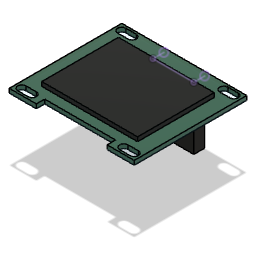
All together (Autodesk Fusion 360 archive; units mm, degrees)
design "oled"
description: IIC OLED 0.96" 4Pin SSD1306
part number: GME12864-11
Autodesk Fusion 360 part; units mm, degrees
sketch "Sketch1" plane through (0, 0, 0) normal (0, 1, 0) x (1, 0, 0)
  line L0 (0, 0) -> (30, 0)
  line L1 (30, 0) -> (30, -27)
  line L2 (30, -27) -> (0, -27)
  line L3 (0, -27) -> (0, 0)
  line L4 (6.5, -27) -> (6.5, -25)
  line L5 (6.5, -25) -> (23.5, -25)
  line L6 (23.5, -25) -> (23.5, -27)
  line L7 (15, -27) -> (15, -25) construction
  line L8 (3.5, -4.3) -> (26.5, -4.3)
  line L9 (26.5, -4.3) -> (26.5, -22.7)
  line L10 (26.5, -22.7) -> (3.5, -22.7)
  line L11 (3.5, -22.7) -> (3.5, -4.3)
  line L12 (1.5, -2.5) -> (4, -2.5)
  arc A0 (4, -2.5) -> (4, -0.5) centre (4, -1.5) ccw
  line L13 (4, -0.5) -> (1.5, -0.5)
  arc A1 (1.5, -0.5) -> (1.5, -2.5) centre (1.5, -1.5) ccw
  line L14 (1.5, -1.5) -> (4, -1.5) construction
  line L15 (15, 0) -> (15, -25) construction
  line L16 (0, -13.5) -> (30, -13.5) construction
  arc A2 (26, -0.5) -> (26, -2.5) centre (26, -1.5) ccw
  line L17 (26, -0.5) -> (28.5, -0.5)
  arc A3 (28.5, -2.5) -> (28.5, -0.5) centre (28.5, -1.5) ccw
  line L18 (28.5, -2.5) -> (26, -2.5)
  line L19 (26, -26.5) -> (28.5, -26.5)
  arc A4 (28.5, -26.5) -> (28.5, -24.5) centre (28.5, -25.5) ccw
  line L20 (28.5, -24.5) -> (26, -24.5)
  arc A5 (26, -24.5) -> (26, -26.5) centre (26, -25.5) ccw
  line L21 (4, -26.5) -> (1.5, -26.5)
  arc A6 (4, -26.5) -> (4, -24.5) centre (4, -25.5) ccw
  arc A7 (1.5, -24.5) -> (1.5, -26.5) centre (1.5, -25.5) ccw
  line L22 (1.5, -24.5) -> (4, -24.5)
  dimension "d1" = 30
  dimension "d2" = 27
  dimension "d3" = 6.5
  dimension "d4" = 2
  dimension "d5" = 3.5
  dimension "d6" = 3.5
  dimension "d7" = 4.3
  dimension "d8" = 4.3
  dimension "d22" = 1.5
  dimension "d23" = 1.5
  dimension "d24" = 1
  dimension "d25" = 2.5
  constraint horizontal L0
  constraint vertical L1
  constraint horizontal L2
  constraint vertical L3
  constraint coincident L0.start L3.end
  constraint coincident L2 L4.start
  constraint perpendicular L2 L4
  constraint perpendicular L4 L5
  constraint coincident L2 L6.end
  constraint perpendicular L2 L6
  constraint midpoint L2 L7.start
  constraint midpoint L5 L7.end
  constraint perpendicular L2 L7
  constraint horizontal L8
  constraint vertical L9
  constraint horizontal L10
  constraint vertical L11
  constraint tangent L12 A0
  constraint tangent A0 L13
  constraint parallel L12 L13
  constraint tangent L13 A1
  constraint tangent L12 A1
  constraint horizontal L14
  constraint midpoint L0 L15.start
  constraint midpoint L3 L16.start
  constraint midpoint L1 L16.end
  constraint symmetric L12.start L15 A3.start
  constraint symmetric L12.end L15 A2.end
  constraint symmetric A0.end L15 A2.start
  constraint symmetric L13.end L15 L17.end
  constraint symmetric A0 L15 A2
  constraint symmetric A1 L15 A3
  constraint symmetric L12.start L16 A7.start
  constraint symmetric L12.end L16 A6.end
  constraint symmetric A0.end L16 L21.start
  constraint symmetric L13.end L16 L21.end
  constraint symmetric A0 L16 A6
  constraint symmetric A1 L16 A7
  constraint symmetric L16 A2.end L20.end
  constraint symmetric L16 A2.start L19.start
  constraint symmetric L16 A2 A5
  constraint symmetric L16 L17.end L19.end
  constraint symmetric L16 A3.start A4.end
  constraint symmetric L16 A3 A4
  measures "d1" distance of L0.start L0.end
  measures "d2" distance of L0.start L2.end
  measures "d3" distance of L1 L6
  measures "d4" distance of L2 L5
  measures "d5" distance of L1 L9
  measures "d6" distance of L3 L11
  measures "d7" distance of L0 L8
  measures "d8" distance of L2 L10
  measures "d22" distance of L3 A1.centre
  measures "d23" distance of L0 A1.centre
  measures "d24" radius of A1
  measures "d25" distance of A1.centre A0.centre
extrude "Extrude1" add sketch "Sketch1" along normal blind 1 contours L8 L9 L10 L11 makes body 1
extrude "Extrude2" add sketch "Sketch1" against normal blind 1 separate body contours L0 L1 L2 L3 L4 L5 L6 | L8 L9 L10 L11 makes body 2
sketch "Sketch2" plane through (0, -1, 0) normal (0, -1, 0) x (1, 0, 0)
  line L0 (6.5, 25) -> (6.5, 27)
  line L1 (6.5, 27) -> (0, 27)
  line L2 (0, 27) -> (0, 0)
  line L3 (0, 0) -> (30, 0)
  line L4 (30, 0) -> (30, 27)
  line L5 (30, 27) -> (23.5, 27)
  line L6 (23.5, 27) -> (23.5, 25)
  line L7 (23.5, 25) -> (6.5, 25)
  line L8 (10.1, 2.6) -> (19.9, 2.6)
  line L9 (19.9, 2.6) -> (19.9, 0)
  line L10 (10.1, 0) -> (10.1, 2.6)
  line L11 (15, 0) -> (15, 2.6) construction
  arc A0 (26, 2.5) -> (26, 0.5) centre (26, 1.5) ccw
  line L12 (26, 2.5) -> (28.5, 2.5)
  arc A1 (28.5, 0.5) -> (28.5, 2.5) centre (28.5, 1.5) ccw
  line L13 (28.5, 0.5) -> (26, 0.5)
  arc A2 (26, 26.5) -> (26, 24.5) centre (26, 25.5) ccw
  line L14 (26, 26.5) -> (28.5, 26.5)
  arc A3 (28.5, 24.5) -> (28.5, 26.5) centre (28.5, 25.5) ccw
  line L15 (28.5, 24.5) -> (26, 24.5)
  arc A4 (4, 24.5) -> (4, 26.5) centre (4, 25.5) ccw
  line L16 (4, 24.5) -> (1.5, 24.5)
  arc A5 (1.5, 26.5) -> (1.5, 24.5) centre (1.5, 25.5) ccw
  line L17 (1.5, 26.5) -> (4, 26.5)
  arc A6 (1.5, 2.5) -> (1.5, 0.5) centre (1.5, 1.5) ccw
  line L18 (1.5, 2.5) -> (4, 2.5)
  arc A7 (4, 0.5) -> (4, 2.5) centre (4, 1.5) ccw
  line L19 (4, 0.5) -> (1.5, 0.5)
  dimension "d13" = 9.8
  dimension "d14" = 2.6
  constraint horizontal L8
  constraint vertical L9
  constraint vertical L10
  constraint midpoint L3 L11.start
  constraint perpendicular L3 L11
  constraint coincident L3 L9.end
  constraint coincident L3 L10.start
  constraint midpoint L8 L11.end
  measures "d13" distance of L8.start L8.end
  measures "d14" distance of L8.start L10.start
extrude "Extrude3" add sketch "Sketch2" along normal blind 15 separate body contours L3 L8 L9 L10 makes body 3
sketch "Minimal Projection" plane through (0, -1, 0) normal (0, -1, 0) x (1, 0, 0)
  arc A0 (26, 2.5) -> (26, 0.5) centre (26, 1.5) ccw
  line L0 (26, 2.5) -> (28.5, 2.5)
  arc A1 (28.5, 0.5) -> (28.5, 2.5) centre (28.5, 1.5) ccw
  line L1 (28.5, 0.5) -> (26, 0.5)
  arc A2 (26, 26.5) -> (26, 24.5) centre (26, 25.5) ccw
  line L2 (26, 26.5) -> (28.5, 26.5)
  arc A3 (28.5, 24.5) -> (28.5, 26.5) centre (28.5, 25.5) ccw
  line L3 (28.5, 24.5) -> (26, 24.5)
  arc A4 (4, 24.5) -> (4, 26.5) centre (4, 25.5) ccw
  line L4 (4, 24.5) -> (1.5, 24.5)
  arc A5 (1.5, 26.5) -> (1.5, 24.5) centre (1.5, 25.5) ccw
  line L5 (1.5, 26.5) -> (4, 26.5)
  arc A6 (1.5, 2.5) -> (1.5, 0.5) centre (1.5, 1.5) ccw
  line L6 (1.5, 2.5) -> (4, 2.5)
  arc A7 (4, 0.5) -> (4, 2.5) centre (4, 1.5) ccw
  line L7 (4, 0.5) -> (1.5, 0.5)
  line L8 (6.5, 25) -> (6.5, 27)
  line L9 (6.5, 27) -> (0, 27)
  line L10 (0, 27) -> (0, 0)
  line L11 (0, 0) -> (30, 0)
  line L12 (30, 0) -> (30, 27)
  line L13 (30, 27) -> (23.5, 27)
  line L14 (23.5, 27) -> (23.5, 25)
  line L15 (23.5, 25) -> (6.5, 25)
  line L16 (19.9, 0) -> (19.9, 2.6)
  line L17 (19.9, 2.6) -> (10.1, 2.6)
  line L18 (10.1, 2.6) -> (10.1, 0)

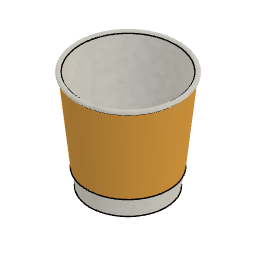
design "Cup"
Autodesk Fusion 360 part; units mm, degrees
sketch "Sketch3" plane through (0, 0, 0) normal (0, 1, 0) x (1, 0, 0)
  line L0 (0, 0) -> (22.3917, 0)
  line L1 (29, -54.5) -> (22.5, 5.5)
  line L2 (0, 5.5) -> (0, -54.5)
  line L3 (21.7959, 5.5) -> (28.2959, -54.5)
  line L4 (28.2959, -54.5) -> (29, -54.5)
  line L5 (21.7959, 5.5) -> (22.5, 5.5)
  line L6 (0, -0.7) -> (22.4676, -0.7)
  circle A0 centre (29.4178, -53.25) radius 1.25
  line L7 (29, -54.5) -> (29.4178, -54.5)
  line L8 (29.4333, -52.0001) -> (24.3174, -4.7764)
  line L9 (24.3174, -4.7764) -> (23.6214, -4.8518)
  arc A1 (22.5338, 5.1877) -> (21.8379, 5.1123) centre (22.1859, 5.15) ccw
  dimension "d4" = 60
  dimension "d5" = 58
  dimension "d6" = 45
  dimension "d7" = 5.5
  dimension "d9" = 0.7
  dimension "d10" = 0.7
  dimension "d11" = 2.5
  dimension "d12" = 47.5
  dimension "d13" = 0.7
  constraint coincident L0.start origin
  constraint horizontal L0
  constraint perpendicular L0 L2
  constraint coincident L0.start L2
  constraint horizontal L1.end L2.start
  constraint horizontal L1.start L2.end
  constraint horizontal L5
  constraint horizontal L4
  constraint coincident L0.end L3
  constraint parallel L1 L3
  constraint coincident L2 L6.start
  constraint coincident L3 L6.end
  constraint perpendicular L2 L6
  constraint tangent L3 A0
  constraint tangent L4 A0
  constraint coincident A0 L7.end
  constraint tangent A0 L7
  constraint coincident A0 L8.start
  constraint parallel L1 L8
  constraint coincident L1 L9.end
  constraint perpendicular L1 L9
  constraint coincident L3 A1.end
  constraint coincident L1 A1.start
  constraint tangent L1 A1
  constraint tangent L3 A1
  constraint tangent L5 A1
  measures "d4" distance of L2.start L2.end
  measures "d7" distance of L0 L5
  measures "d9" distance of L1 L3
  measures "d10" distance of L0 L6
  measures "d11" diameter of A0
  measures "d12" distance of L8.start L8.end
  measures "d13" distance of L8.end L9.end
revolve "Revolve1" add sketch "Sketch3" angle 360 about axis through (0, 0, -5.5) along (0, 0, 1) contours L0 L2 L3 L6 | L1 L3 A0 A1 | L1 A0 | L1 A0 makes body 1
revolve "Revolve2" add sketch "Sketch3" angle 360 about axis through (0, 0, -5.5) along (0, 0, 1) separate body contours L1 A0 L8 L9 makes body 2
equation "d10 = d9"

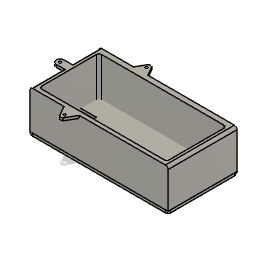
design "Sensor Housing"
Autodesk Fusion 360 part; units mm, degrees
sketch "Outside box sketch" plane through (0, 0, 0) normal (0, 0, 1) x (1, 0, 0)
  line L0 (1, 0) -> (52, 0)
  line L1 (53, 1) -> (53, 14.9)
  line L2 (52, 15.9) -> (1, 15.9)
  line L3 (0, 14.9) -> (0, 1)
  arc A0 (1, 15.9) -> (0, 14.9) centre (1, 14.9) ccw
  arc A1 (0, 1) -> (1, 0) centre (1, 1) ccw
  arc A2 (53, 14.9) -> (52, 15.9) centre (52, 14.9) ccw
  arc A3 (52, 0) -> (53, 1) centre (52, 1) ccw
  point P0 (53, 0)
  point P1 (0, 15.9)
  dimension "d1" = 53
  dimension "d2" = 15.9
  dimension "d13" = 1
  dimension "d14" = 1
  dimension "d15" = 1
  dimension "d16" = 1
  constraint horizontal L0
  constraint vertical L1
  constraint horizontal L2
  constraint vertical L3
  constraint coincident P1 L2
  constraint coincident P1 L3
  constraint tangent L2 A0
  constraint tangent L3 A0
  constraint coincident origin L0
  constraint coincident origin L3
  constraint tangent L0 A1
  constraint tangent L3 A1
  constraint tangent L2 A2
  constraint tangent L1 A2
  constraint coincident P0 L0
  constraint coincident P0 L1
  constraint tangent L0 A3
  constraint tangent L1 A3
  measures "d1" distance of origin P0
  measures "d2" distance of origin P1
  measures "d13" radius of A0
  measures "d14" radius of A1
  measures "d15" radius of A2
  measures "d16" radius of A3
extrude "Extrude1" add sketch "Outside box sketch" along normal blind 26.5 makes body 1
sketch "Hole sketch" plane through (0, 0, 0) normal (0, 1, 0) x (1, 0, 0)
  line L0 (3, -2) -> (50, -2)
  line L1 (51, -3) -> (51, -24)
  line L2 (50, -25) -> (3, -25)
  line L3 (2, -24) -> (2, -3)
  arc A0 (3, -2) -> (2, -3) centre (3, -3) ccw
  arc A1 (51, -3) -> (50, -2) centre (50, -3) ccw
  arc A2 (50, -25) -> (51, -24) centre (50, -24) ccw
  arc A3 (2, -24) -> (3, -25) centre (3, -24) ccw
  dimension "d17" = 1
  constraint horizontal L0
  constraint vertical L1
  constraint horizontal L2
  constraint vertical L3
  constraint tangent L0 A0
  constraint tangent L3 A0
  constraint tangent L0 A1
  constraint tangent L1 A1
  constraint equal A0 A1
  constraint tangent L1 A2
  constraint tangent L2 A2
  constraint equal A0 A2
  constraint tangent L2 A3
  constraint tangent L3 A3
  constraint equal A0 A3
  measures "d17" radius of A0
extrude "Extrude2" cut sketch "Hole sketch" along normal blind 25 bodies 1
sketch "Base sketch" plane through (0, 0, 0) normal (0, 1, 0) x (1, 0, 0)
  line L0 (1, 0) -> (52, 0)
  line L1 (53, -1) -> (53, -25.5)
  line L2 (52, -26.5) -> (1, -26.5)
  arc A0 (1, 0) -> (0, -1) centre (1, -1) ccw
  arc A1 (53, -1) -> (52, 0) centre (52, -1) ccw
  arc A2 (52, -26.5) -> (53, -25.5) centre (52, -25.5) ccw
  arc A3 (0, -25.5) -> (1, -26.5) centre (1, -25.5) ccw
  line L3 (0, -1) -> (0, -25.5)
  line L4 (1, -9) -> (8, -9)
  line L5 (8, -9) -> (8, -18)
  line L6 (8, -18) -> (1, -18)
  line L7 (1, -18) -> (1, -9)
  line L8 (1, -9) -> (8, -9)
  line L9 (1, -9) -> (8, -9)
  line L10 (8, -9) -> (8, -18)
  line L11 (45, -9) -> (45, -18)
  line L12 (52, -9) -> (45, -9)
  line L13 (52, -18) -> (52, -9)
  line L14 (45, -18) -> (52, -18)
  point P0 (53, 0)
  point P1 (0, -26.5)
  constraint horizontal L0
  constraint vertical L1
  constraint horizontal L2
  constraint coincident origin L0
  constraint tangent L0 A0
  constraint coincident P0 L0
  constraint coincident P0 L1
  constraint tangent L0 A1
  constraint tangent L1 A1
  constraint tangent L1 A2
  constraint tangent L2 A2
  constraint equal A1 A2
  constraint coincident P1 L2
  constraint tangent L2 A3
  constraint equal A1 A3
  constraint vertical L3
  constraint horizontal L4
  constraint vertical L5
  constraint horizontal L6
  constraint vertical L7
  constraint horizontal L8
  constraint horizontal L9
  constraint vertical L10
extrude "Extrude3" add sketch "Base sketch" along normal blind 1 separate body contours L0 L1 L2 A0 A1 A2 A3 L3 | L4 L5 L6 L7 L8 L9 L10 | L11 L12 L13 L14 makes body 2
extrude "Extrude4" cut sketch "Base sketch" along normal blind 26 contours L0 L1 L2 A0 A1 A2 A3 L3 | L4 L5 L6 L7 L8 L9 L10 | L11 L12 L13 L14 bodies 2
extrude "Extrude5" add sketch "Base sketch" along normal blind 1 bodies 2
sketch "Front hole sketch" plane through (0, 0, 0) normal (0, 1, 0) x (1, 0, 0)
  line L0 (-2.4094, -14) -> (0, -14)
  line L1 (0, -14) -> (0, -11)
  line L2 (0, -11) -> (-2.4095, -11)
  arc A0 (-2.4095, -11) -> (-2.4094, -14) centre (-2.4095, -12.5) ccw
  circle A1 centre (-2.4095, -12.5) radius 0.5
  dimension "d24" = 1
  constraint horizontal L0
  constraint vertical L1
  constraint horizontal L2
  constraint concentric A0 A1
  measures "d24" diameter of A1
extrude "Extrude6" add sketch "Front hole sketch" along normal blind 13.9 separate body makes body 3
extrude "Extrude7" cut 1 faces at (-0.6365, 0, 12.5) along direction (0, 1, 0) blind 12.9 on bodies 3 bodies 3
sketch "Side holes sketch" plane through (0, 0, 0) normal (0, 1, 0) x (1, 0, 0)
  line L0 (13.1017, 0.0509) -> (19, 0.0509) construction
  line L1 (13.1017, 0.0509) -> (18.8983, 0.0509)
  line L2 (13.1017, -26.6022) -> (18.8983, -26.6022)
  line L3 (13.1017, -26.6022) -> (15.3819, -30.5516)
  line L4 (16, -31.6222) -> (16.1017, -31.7984)
  line L5 (18.8983, -26.6022) -> (16.6709, -30.4601)
  line L6 (16, -31.6222) -> (15.8983, -31.7984)
  arc A0 (15.3819, -30.5516) -> (16.6709, -30.4601) centre (15.9305, -29.1556) ccw
  circle A1 centre (15.9305, -29.1556) radius 0.5
  line L7 (18.7811, -0.0196) -> (16.6709, 3.6353)
  line L8 (13.2189, -0.0196) -> (15.3819, 3.7269)
  line L9 (13.2189, -0.0196) -> (18.7811, -0.0196)
  arc A2 (16.6709, 3.6353) -> (15.3819, 3.7269) centre (15.9305, 2.3308) ccw
  circle A3 centre (15.9305, 2.3308) radius 0.5
  point P0 (15.9305, 2.3308)
  dimension "d32" = 1
  dimension "d33" = 1
  constraint horizontal L0
  constraint coincident L4.start L5
  constraint collinear L3 L4
  constraint collinear L5 L6
  constraint concentric A0 A1
  constraint concentric A2 A3
  measures "d32" diameter of A1
  measures "d33" diameter of A3
extrude "Extrude8" add sketch "Side holes sketch" along normal blind 13.9 separate body contours L1 L7 L8 A2 | L2 L3 L5 A0 makes body 4 at (15.0865, 4.6333, -0.0509) makes body 5 at (15.0339, 4.6333, 26.6022)
extrude "Extrude9" cut 2 faces at (15.9893, 0, 27.2871) (15.9893, 0, -0.6446) along direction (0, 1, 0) blind 12.9 on bodies 4 5 bodies 4 5
extrude "Extrude10" add 2 faces at (15.9893, 13.9, 27.2871) (15.9893, 13.9, -0.6446) along direction (0, 1, 0) blind 2 on bodies 4 5 bodies 5 4
extrude "Extrude11" cut 2 faces at (15.9893, 12.9, 27.2871) (15.9893, 12.9, -0.6446) along direction (0, 1, 0) blind 2 on bodies 4 5 bodies 4 5
extrude "Extrude12" add 1 faces at (-0.6365, 13.9, 12.5) along direction (0, 1, 0) blind 2 on bodies 3 bodies 1 2 3
extrude "Extrude13" cut 1 faces at (-0.6365, 12.9, 12.5) along direction (0, 1, 0) blind 2 on bodies 1 bodies 1
extrude "Extrude14" add 1 faces at (0, 15.2333, 13) along direction (1, 0, 0) blind 1 on bodies 1 bodies 1
extrude "Extrude15" add 1 faces at (15.0865, 15.2333, -0.0509) along direction (0, 0, 1) blind 2 on bodies 4 bodies 1 4
extrude "Extrude16" add 1 faces at (15.0339, 15.2333, 26.6022) along direction (0, 0, -1) blind 1.6 on bodies 5 bodies 1 5
named bodies: "Outside box", "Base", "Front hole", "Side hole 1", "Side hole 2"

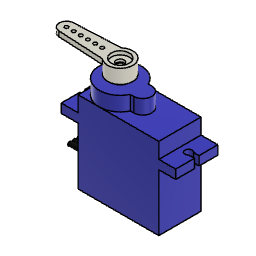
design "SG90 Micro Servo"
Autodesk Fusion 360 part; units mm, degrees
sketch "Sketch2" plane through (0, 0, 0) normal (0, 1, 0) x (1, 0, 0)
  line L0 (0, 0) -> (22.5, 0)
  line L1 (22.5, 0) -> (22.5, -22.75)
  line L2 (22.5, -22.75) -> (0, -22.75)
  line L3 (0, -22.75) -> (0, 0)
  line L4 (-4.7, -15.9) -> (-4.7, -18.4)
  line L5 (27.2, -18.4) -> (27.2, -15.9)
  line L6 (-4.7, -18.4) -> (0, -18.4)
  line L7 (22.5, -18.4) -> (27.2, -18.4)
  line L8 (27.2, -15.9) -> (22.5, -15.9)
  line L9 (0, -15.9) -> (-4.7, -15.9)
  dimension "d3" = 22.5
  dimension "d4" = 22.75
  dimension "d6" = 4.35
  dimension "d7" = 2.5
  dimension "d8" = 4.7
  dimension "d9" = 4.7
  constraint horizontal L0
  constraint vertical L1
  constraint horizontal L2
  constraint vertical L3
  constraint coincident L0.start L3.end
  constraint horizontal L8
  constraint vertical L4
  constraint horizontal L6
  constraint vertical L5
  constraint coincident L3 L6.end
  constraint coincident L1 L7.start
  constraint collinear L6 L7
  constraint coincident L1 L8.end
  constraint coincident L3 L9.start
  constraint collinear L8 L9
  measures "d3" distance of L0.start L0.end
  measures "d4" distance of L0.start L2.end
  measures "d6" distance of L2 L6
  measures "d7" distance of L5.end L5.start
  measures "d8" distance of L1 L5
  measures "d9" distance of L3 L4
extrude "Extrude2" add sketch "Sketch2" along normal blind 11.75 makes body 1
sketch "Sketch3" plane through (0, 0, 22.75) normal (0, 0, 1) x (-1, 0, 0)
  line L0 (0, 0) -> (-22.5, 0)
  line L1 (-22.5, 0) -> (-22.5, -11.75)
  line L2 (-22.5, -11.75) -> (0, -11.75)
  line L3 (0, -11.75) -> (0, 0)
  circle A0 centre (-5.875, -5.875) radius 5.875
  line L4 (-5.875, -5.875) -> (-12.175, -5.875) construction
  line L5 (-11.1915, -8.375) -> (-12.175, -8.375)
  line L6 (-11.1915, -3.375) -> (-12.175, -3.375)
  arc A1 (-12.175, -3.375) -> (-12.175, -8.375) centre (-12.175, -5.875) ccw
  dimension "d13" = 6.3
  dimension "d14" = 2.5
  constraint tangent L0 A0
  constraint tangent L2 A0
  constraint tangent L3 A0
  constraint coincident A0.centre L4.start
  constraint coincident L4.end A1.centre
  constraint horizontal L4
  constraint coincident A0 L5.start
  constraint tangent L5 A1
  constraint coincident A0 L6.start
  constraint tangent L6 A1
  constraint horizontal L5
  constraint horizontal L6
  measures "d13" distance of A0.centre L4.end
  measures "d14" radius of A1
extrude "Extrude3" add sketch "Sketch3" along normal blind 4 contours A0 | A0 L5 L6 A1 bodies 1
sketch "Sketch4" plane through (0, 0, 26.75) normal (0, 0, 1) x (-1, 0, 0)
  arc A0 (-11.1915, -8.375) -> (-11.1915, -3.375) centre (-5.875, -5.875) ccw
  line L0 (-11.1915, -3.375) -> (-12.175, -3.375)
  arc A1 (-12.175, -3.375) -> (-12.175, -8.375) centre (-12.175, -5.875) ccw
  line L1 (-12.175, -8.375) -> (-11.1915, -8.375)
  circle A2 centre (-5.875, -5.875) radius 2.3
  circle A3 centre (-5.875, -5.875) radius 0.75
  dimension "d17" = 4.6
  dimension "d28" = 1.5
  constraint concentric A0 A2
  constraint concentric A2 A3
  measures "d17" diameter of A2
  measures "d28" diameter of A3
extrude "Extrude4" add sketch "Sketch4" along normal blind 3.15 separate body contours A2 makes body 2
sketch "Sketch5" plane through (0, 0, 18.4) normal (0, 0, 1) x (-1, 0, 0)
  line L0 (4.7, 0) -> (0, 0)
  line L1 (0, 0) -> (0, -11.75)
  line L2 (0, -11.75) -> (4.7, -11.75)
  line L3 (4.7, -11.75) -> (4.7, 0)
  line L4 (-22.5, 0) -> (-27.2, 0)
  line L5 (-27.2, 0) -> (-27.2, -11.75)
  line L6 (-27.2, -11.75) -> (-22.5, -11.75)
  line L7 (-22.5, -11.75) -> (-22.5, 0)
  line L8 (-27.2, -5.875) -> (4.7, -5.875) construction
  line L9 (-11.25, -5.875) -> (-11.25, -0.3179)
  line L10 (4.7, -6.525) -> (3.1599, -6.525)
  line L11 (4.7, -5.225) -> (3.1599, -5.225)
  arc A0 (3.1599, -5.225) -> (3.1599, -6.525) centre (2.4, -5.875) ccw
  arc A1 (-25.6599, -6.525) -> (-25.6599, -5.225) centre (-24.9, -5.875) ccw
  line L12 (-27.2, -5.225) -> (-25.6599, -5.225)
  line L13 (-27.2, -6.525) -> (-25.6599, -6.525)
  dimension "d20" = 2
  dimension "d21" = 1.3
  dimension "d22" = 2.3
  constraint midpoint L5 L8.start
  constraint midpoint L3 L8.end
  constraint midpoint L8 L9.start
  constraint perpendicular L8 L9
  constraint coincident L8 A0.centre
  constraint coincident L3 L10.start
  constraint perpendicular L3 L10
  constraint coincident L3 L11.start
  constraint perpendicular L3 L11
  constraint symmetric L8 L10 L11
  constraint symmetric L9 L10.start L13.start
  constraint symmetric L9 L10.end A1.start
  constraint symmetric L9 L11.start L12.start
  constraint symmetric L9 L11.end A1.end
  constraint symmetric L9 A0 A1
  measures "d20" diameter of A0
  measures "d21" distance of L10 L11
  measures "d22" distance of L3 A0.centre
extrude "Extrude5" cut sketch "Sketch5" against normal through all contours L3 L10 L11 A0 | L5 A1 L12 L13 bodies 1
sketch "Sketch6" plane through (0, 0, 0) normal (-1, 0, 0) x (0, -1, 0)
  line L0 (0, 0) -> (0, 15.9)
  line L1 (0, 15.9) -> (-11.75, 15.9)
  line L2 (-11.75, 15.9) -> (-11.75, 0)
  line L3 (-11.75, 0) -> (0, 0)
  line L4 (-4.075, 5.7) -> (-7.675, 5.7) construction
  line L5 (-7.675, 5.7) -> (-7.675, 4.5) construction
  line L6 (-7.675, 4.5) -> (-4.075, 4.5) construction
  line L7 (-4.075, 4.5) -> (-4.075, 5.7) construction
  line L8 (-5.875, 4.5) -> (-5.875, 0) construction
  circle A0 centre (-5.875, 5.1) radius 0.6
  circle A1 centre (-4.675, 5.1) radius 0.6
  circle A2 centre (-7.075, 5.1) radius 0.6
  dimension "d24" = 1.2
  dimension "d25" = 4.5
  constraint horizontal L4
  constraint vertical L5
  constraint horizontal L6
  constraint vertical L7
  constraint midpoint L6 L8.start
  constraint coincident L3 L8.end
  constraint perpendicular L3 L8
  constraint midpoint L3 L8.end
  constraint tangent L4 A0
  constraint coincident L8.start A0
  constraint tangent L4 A1
  constraint tangent L7 A1
  constraint tangent L6 A1
  constraint tangent L4 A2
  constraint tangent L5 A2
  constraint tangent L6 A2
  constraint tangent A0 A1
  constraint tangent A0 A2
  measures "d24" distance of L4.start L6.end
  measures "d25" distance of L8.start L8.end
extrude "Extrude6" add sketch "Sketch6" along normal blind 7 separate body contours A0 | A2 | A1 makes body 3
sketch "Sketch1" plane through (0, 0, 29.9) normal (0, 0, 1) x (-1, 0, 0) in component "Horn"
  circle A0 centre (-5.875, -5.875) radius 0.75
  circle A1 centre (-5.875, -5.875) radius 2.3
  circle A2 centre (-5.875, -5.875) radius 3.5
  circle A3 centre (-5.875, -5.875) radius 2.5
  line L0 (-3.5886, -8.525) -> (9.2267, -7.8724)
  line L1 (-3.5886, -3.225) -> (9.2267, -3.8776)
  arc A4 (9.2267, -7.8724) -> (9.2267, -3.8776) centre (9.125, -5.875) ccw
  line L2 (-5.875, -5.875) -> (9.125, -5.875) construction
  circle A5 centre (9.125, -5.875) radius 0.5
  circle A6 centre (7.125, -5.875) radius 0.5
  circle A7 centre (5.125, -5.875) radius 0.5
  circle A8 centre (3.125, -5.875) radius 0.5
  circle A9 centre (1.125, -5.875) radius 0.5
  circle A10 centre (-0.875, -5.875) radius 0.5
  circle A11 centre (-5.875, -5.875) radius 1.1
  dimension "d29" = 7
  dimension "d30" = -1
  dimension "d32" = 2
  dimension "d33" = 5.3
  dimension "d34" = 1
  dimension "d37" = -10
  dimension "d38" = 0
  dimension "d39" = 15
  dimension "d42" = 2.2
  constraint concentric A0 A2
  constraint coincident A2 L0.start
  constraint coincident A2 L1.start
  constraint tangent L0 A4
  constraint tangent L1 A4
  constraint coincident A0.centre A1.centre
  constraint coincident A4.centre L2.end
  constraint horizontal L2
  constraint symmetric L0.start L1.start L2
  constraint concentric A4 A5
  constraint concentric A2 A11
  measures "d29" diameter of A2
  measures "d32" radius of A4
  measures "d33" vertical distance of L0.start L1.start
  measures "d34" diameter of A5
  measures "d39" distance of A0.centre A4.centre
  measures "d42" diameter of A11
extrude "Extrude1" add sketch "Sketch1" against normal blind 2.2 separate body contours A2 | A3 makes body 4 in component "Horn"
extrude "Extrude2'" add sketch "Sketch1" along normal blind 1.7 contours A2 bodies 4 in component "Horn"
extrude "Extrude3'" add sketch "Sketch1" against normal blind 1.4 from surface at 1.7 contours A2 L0 L1 A4 bodies 4 in component "Horn"
extrude "Extrude4'" add sketch "Sketch1" along normal up to surface (0.7 mm away) contours A1 | A3 bodies 4 in component "Horn"
component "Horn" placed x (1, 0, 0) y (0, 1, 0) z (0, 0, 1) at (0, 0, 0)
equation "d43 = 3.9 mm - 2.2 mm"
named bodies: "Body", "Wires", "Mount"

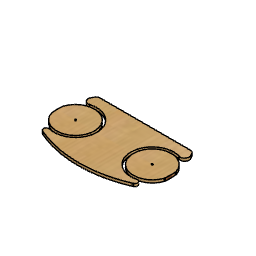
design "Cup Holder"
Autodesk Fusion 360 part; units mm, degrees
sketch "Sketch1" plane through (0, 0, 3) normal (0, 0, 1) x (-1, 0, 0)
  line L0 (27.1642, 47.5117) -> (28.8849, 49.9691)
  line L1 (28.8849, 49.9691) -> (37.0764, 44.2334)
  line L2 (37.0764, 44.2334) -> (35.3557, 41.7759)
  line L3 (35.3557, 41.7759) -> (27.1642, 47.5117)
  line L4 (-28.8849, 49.9691) -> (-27.1642, 47.5117)
  line L5 (-27.1642, 47.5117) -> (-35.3557, 41.7759)
  line L6 (-35.3557, 41.7759) -> (-37.0764, 44.2334)
  line L7 (-37.0764, 44.2334) -> (-28.8849, 49.9691)
  circle A0 centre (0, 0) radius 62.5
  line L8 (-45, -37.5) -> (-45, -34.5)
  line L9 (-45, -34.5) -> (-27, -34.5)
  line L10 (-27, -34.5) -> (-27, -37.5)
  line L11 (-27, -37.5) -> (-45, -37.5)
  line L12 (-9, -37.5) -> (-9, -34.5)
  line L13 (-9, -34.5) -> (9, -34.5)
  line L14 (9, -34.5) -> (9, -37.5)
  line L15 (9, -37.5) -> (-9, -37.5)
  line L16 (27, -37.5) -> (27, -34.5)
  line L17 (27, -34.5) -> (45, -34.5)
  line L18 (45, -34.5) -> (45, -37.5)
  line L19 (45, -37.5) -> (27, -37.5)
  circle A1 centre (-42.2822, 0) radius 21.8379 construction
  circle A2 centre (-42.2822, 0) radius 22.5338 construction
  circle A3 centre (-42.2822, 0) radius 20.8379
  circle A4 centre (-42.2822, 0) radius 23.5338
  line L20 (-45, -34.5) -> (-50, -34.5)
  line L21 (-50, -34.5) -> (-45, -34.5)
  line L22 (-45, -34.5) -> (-27, -34.5)
  line L23 (-27, -34.5) -> (-9, -34.5)
  line L24 (-9, -34.5) -> (9, -34.5)
  line L25 (9, -34.5) -> (27, -34.5)
  line L26 (27, -34.5) -> (45, -34.5)
  line L27 (45, -34.5) -> (50, -34.5)
  line L28 (50, -34.5) -> (45, -34.5)
  line L29 (45, -34.5) -> (27, -34.5)
  line L30 (27, -34.5) -> (9, -34.5)
  line L31 (9, -34.5) -> (-9, -34.5)
  line L32 (-9, -34.5) -> (-27, -34.5)
  line L33 (-27, -34.5) -> (-45, -34.5)
  arc A5 (-53.2887, -32.6583) -> (-50, -34.5) centre (-50, -30.6429) ccw
  arc A6 (50, -34.5) -> (53.2887, -32.6583) centre (50, -30.6429) ccw
  arc A7 (49.0193, 28.9228) -> (-49.0193, 28.9228) centre (0, -86.0646) ccw
  arc A8 (-49.0193, 28.9228) -> (-60.5532, 15.4777) centre (-41.1762, 10.5248) ccw
  arc A9 (60.5532, 15.4777) -> (49.0193, 28.9228) centre (41.1762, 10.5248) ccw
  line L34 (0, 0) -> (0, -86.0646) construction
  line L35 (-43.5472, 36.0401) -> (-35.3557, 41.7759) construction
  circle A10 centre (42.2822, 0) radius 23.5338
  circle A11 centre (42.2822, 0) radius 20.8379
  circle A12 centre (-42.2822, 0) radius 1
  circle A13 centre (42.2822, 0) radius 1
  line L36 (-39.2873, -34.5) -> (-36.1123, -34.5)
  line L37 (-39.2873, -34.5) -> (-36.1123, -34.5)
  line L38 (37.0397, -34.5) -> (40.2147, -34.5)
  line L39 (37.0397, -34.5) -> (40.2147, -34.5)
  line L40 (-44.5, -34.5) -> (-50, -34.5)
  line L41 (50, -34.5) -> (44.5, -34.5)
  line L42 (42.5, -34.5) -> (44.5, -34.5)
  line L43 (42.5, -34.5) -> (44.5, -34.5)
  line L44 (44.5, -34.5) -> (50, -34.5)
  line L45 (-50, -34.5) -> (-44.5, -34.5)
  line L46 (-44.5, -34.5) -> (-42.5, -34.5)
  line L47 (-44.5, -34.5) -> (-42.5, -34.5)
  dimension "d71" = -1
  dimension "d72" = 1
  dimension "d73" = 125
  dimension "d74" = 20
  dimension "d90" = 2
  dimension "d91" = 2
  constraint coincident L20.end L21.start
  constraint coincident L27.end L28.start
  constraint tangent L28 A6
  constraint tangent A0 A6
  constraint coincident A0 A6.end
  constraint coincident A0 A5.start
  constraint tangent L21 A5
  constraint tangent A0 A5
  constraint tangent A7 A9
  constraint tangent A7 A8
  constraint tangent A0 A8
  constraint tangent A0 A9
  constraint coincident A0 A9.start
  constraint coincident A0 A8.end
  constraint coincident A0.centre L34.start
  constraint coincident A7.centre L34.end
  constraint vertical L34
  constraint tangent A7 L35
  constraint equal A8 A9
  constraint symmetric A3 L34 A11
  constraint symmetric A4 L34 A10
  constraint concentric A1 A12
  constraint concentric A11 A13
  measures "d73" radius of A7
  measures "d74" radius of A8
  measures "d90" diameter of A12
  measures "d91" diameter of A13
extrude "Extrude1" add sketch "Sketch1" along normal blind 3 contours A0 L9 L13 L17 A4 L20 L21 L22 L23 L24 L25 L26 L27 L28 L29 L30 L31 L32 L33 A5 A6 A7 A8 A9 A10 L36 L37 L38 L39 L40 L41 L42 L43 L44 L45 L46 L47 | A0 A11 | A0 A3 picked at (55.5374, 4.5167) picked at (-56.0717, 0) makes body 1 at (0, -19.6162, 3) makes body 2 at (56.0717, 0, 3) makes body 3 at (-56.0717, 0, 3)
fillet "Fillet1" radius 5 6 edges at (60.7844, 14.5434, 4.5) (-60.7844, 14.5434, 4.5) (62.1989, 6.1271, 4.5) (62.1989, -6.1271, 4.5) (-62.1989, -6.1271, 4.5) (-62.1989, 6.1271, 4.5) on bodies 1 2 3
fillet "Fillet1" radius 3 2 edges at (-60.7844, -14.5434, 4.5) (60.7844, -14.5434, 4.5) on bodies 1 2 3

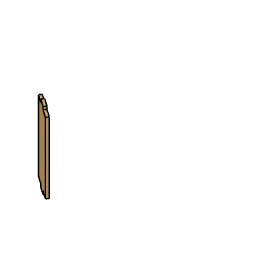
design "Left Support"
Autodesk Fusion 360 part; units mm, degrees
sketch "Sketch1" plane through (0, 0, 3) normal (0, 0, 1) x (-1, 0, 0)
  circle A0 centre (0, 0) radius 62.5
  line L0 (45.2679, 38.4976) -> (43.5472, 36.0401)
  line L1 (43.5472, 36.0401) -> (18.9726, 53.2474)
  line L2 (18.9726, 53.2474) -> (20.6934, 55.7049)
  line L3 (20.6934, 55.7049) -> (45.2679, 38.4976)
  line L4 (0, 0) -> (0, 62.5) construction
  line L5 (35.8485, 51.197) -> (0, 76.2984) construction
  line L6 (35.8485, 51.197) -> (32.9806, 47.1012) construction
  line L7 (35.3557, 41.7759) -> (37.0764, 44.2334)
  line L8 (27.1642, 47.5117) -> (28.8849, 49.9691)
  dimension "d15" = 3
  dimension "d16" = 55
  dimension "d17" = 30
  dimension "d18" = 5
  dimension "d19" = 10
  constraint perpendicular L0 L1
  constraint parallel L0 L2
  constraint parallel L1 L3
  constraint coincident A0.centre L4.start
  constraint coincident A0 L4.end
  constraint vertical L4
  constraint coincident L4 L5.end
  constraint coincident A0 L5.start
  constraint tangent A0 L5
  constraint parallel L3 L5
  constraint midpoint L3 L6.end
  constraint perpendicular L3 L6
  constraint coincident L1 L7.start
  constraint coincident L3 L7.end
  constraint perpendicular L3 L7
  constraint coincident L1 L8.start
  constraint coincident L3 L8.end
  constraint perpendicular L3 L8
  constraint symmetric L6 L7 L8
  measures "d15" distance of L1.end L2.end
  measures "d16" angle of L1 L4
  measures "d17" distance of L0.start L2.end
  measures "d18" distance of L3 L5
  measures "d19" distance of L7 L8
extrude "Extrude1" add sketch "Sketch1" along normal up to surface (78 mm away) and the other way up to surface (3 mm away) contours L1 L3 L7 L8
extrude "Extrude2" add sketch "Sketch1" along normal up to surface (75 mm away) contours L0 L1 L3 L7 | L1 L2 L3 L8

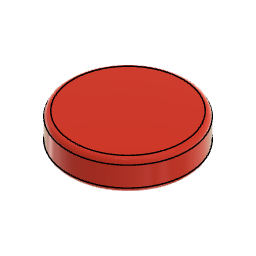
design "Smartie Token"
Autodesk Fusion 360 part; units mm, degrees
sketch "Sketch1" plane through (0, 0, 0) normal (0, 0, 1) x (1, 0, 0)
  circle A0 centre (0, 0) radius 6
  dimension "d1" = 12
  constraint coincident A0.centre origin
  measures "d1" diameter of A0
extrude "Extrude1" add sketch "Sketch1" along normal blind 3
fillet "Fillet1" radius 0.5 2 edges at (-5.594, -2.1697, 0) (-5.594, -2.1697, 3)
